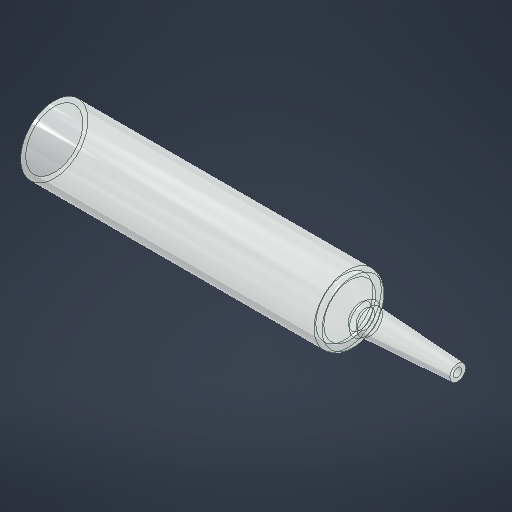
# Autodesk Inventor part: P_Spritze_60ml
Saved by Autodesk Inventor 2026 (Build 300175000, 175)
## iProperties
Created: 2025-04-25
Part Number: P_Spritze_60ml
Material: Glas
Document SubType Name: Modeling
Designer: FAL
Density: 2.18 g/cm^3
Appearance: Klar
Author: FAL
Autodesk Inventor part; units mm, degrees
ref_plane "YZ Plane" through (0, 0, 0) normal (1, 0, 0) x (0, 1, 0)
ref_plane "XZ Plane" through (0, 0, 0) normal (0, 1, 0) x (-1, 0, 0)
ref_plane "XY Plane" through (0, 0, 0) normal (0, 0, 1) x (1, 0, 0)
sketch "Skizze2" plane through (0, 0, 0) normal (0, 0, 1) x (1, 0, 0)
  line L0 (0, 0) -> (52.5603, 0) construction
  line L1 (0, 12.75) -> (0, 15)
  line L2 (0, 15) -> (131.1081, 15)
  line L3 (129.6756, 12.75) -> (0, 12.75)
  line L4 (0, 12.75) -> (0, 0) construction
  line L5 (180.3, 3.5) -> (140.9879, 5.6733)
  line L6 (138.7612, 6.8584) -> (133.5003, 13.8103)
  line L7 (180.3, 3.5) -> (180.2102, 1.875)
  line L8 (180.2102, 1.875) -> (139.0031, 4.153)
  line L9 (136.7765, 5.3381) -> (132.0678, 11.5603)
  arc A0 (133.5003, 13.8103) -> (131.1081, 15) centre (131.1081, 12) ccw
  arc A1 (138.7612, 6.8584) -> (140.9879, 5.6733) centre (141.1534, 8.6687) ccw
  arc A2 (132.0678, 11.5603) -> (129.6756, 12.75) centre (129.6756, 9.75) ccw
  arc A3 (136.7765, 5.3381) -> (139.0031, 4.153) centre (139.1687, 7.1485) ccw
  point P0 (132.6, 15)
  point P1 (131.1675, 12.75)
  point P2 (139.6, 5.75)
  point P3 (137.6153, 4.2298)
  dimension "d2" = 30
  dimension "d4" = 25.5
  dimension "d5" = 7
  dimension "d6" = 3.75
  dimension "d7" = 40.7
  dimension "d8" = 11.5
  dimension "d9" = 7
  dimension "d10" = 2.5
  dimension "d11" = 180.3
  dimension "d12" = 3
  constraints: 20 end point, 8 point on circle, 8 point on line, 8 tangent, 4 centre point, 3 equal radius, 3 perpendicular, 2 parallel, 1 vertical
  measures "d2" diameter of L2 L0
  measures "d4" diameter of L3 L0
  measures "d5" horizontal distance of point (139.6, 5.75) point (132.6, 15)
  measures "d6" diameter of L7.end L0
  measures "d7" horizontal distance of L5.start point (139.6, 5.75)
  measures "d8" diameter of point (139.6, 5.75) L0
  measures "d9" diameter of L5.start L0
  measures "d10" distance between parallel lines of L6 L9
  measures "d11" distance from line of L4 L5.start
  measures "d12" radius of A0
revolve "Umdrehung1" add sketch "Skizze2" angle 360 about axis through (0, 0, 0) along (1, 0, 0)
sketch "Skizze3" plane through (0, 0, 0) normal (-1, 0, 0) x (0, 0, 1)
  circle A0 centre (0, 0) radius 1.875 projected
  arc A1 (0, 12.75) -> (-12.75, 0) centre (0, 0) ccw
  arc A2 (0, 16) -> (-5.7621, 14.9264) centre (0, 0) ccw
  line L0 (0, 0) -> (-25, 0)
  line L1 (-25, 0) -> (-25, 7.5)
  line L2 (-25, 7.5) -> (-5.7621, 14.9264)
  line L3 (0, 0) -> (0, 16)
  circle A3 centre (0, 0) radius 12.75 projected
  dimension "d13" = 25
  dimension "d14" = 16
  dimension "d15" = 7.5
  constraints: 8 end point, 4 point on circle, 2 centre point, 2 coincident, 2 point on line, 1 concentric, 1 horizontal, 1 perpendicular, 1 tangent, 1 vertical
  measures "d13" distance from line of L1 point (0, 0)
  measures "d14" radius of A2
  measures "d15" distance of L0.end L1.end
